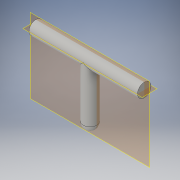
# Autodesk Inventor part: camPost
Saved by Autodesk Inventor 2016 (Build 200138000, 138)
## iProperties
Created: 2015-07-26
Part Number: camPost
Material: Generic
Document SubType Name: Modeling
Designer: steele
Density: 1 g/cm^3
Appearance: Default
Author: steele
Autodesk Inventor part; units mm, degrees
ref_plane "YZ Plane" through (0, 0, 0) normal (1, 0, 0) x (0, 1, 0)
sketch "Sketch1" plane through (0, 0, 0) normal (1, 0, 0) x (0, 1, 0)
  circle A0 centre (0, 0) radius 3.175
  dimension "postHoleDiam" = 6.35
  constraints: 1 centre point, 1 coincident
  measures "postHoleDiam" diameter of A0
extrude "Extrusion1" add sketch "Sketch1" along normal mid plane 50.8
sketch "Sketch3" plane through (0, 0, 0) normal (0, 1, 0) x (-1, 0, 0)
  circle A0 centre (0, 0) radius 3.175
  line L0 (25.4, 3.175) -> (-25.4, 3.175) projected
  constraints: 1 centre point, 1 coincident, 1 tangent
extrude "Extrusion2" add sketch "Sketch3" against normal blind 25.4
ref_plane "Work Plane1" through (0, -31.75, 0) normal (0, -1, 0) x (1, 0, 0)
sketch "Sketch5" plane through (0, 0, 0) normal (0, 0, 1) x (1, 0, 0)
  line L0 (-3.175, -25.4) -> (3.175, -25.4) projected
  arc A0 (-3.175, -25.4) -> (0, -28.575) centre (0, -25.4) ccw
  line L1 (0, -25.4) -> (0, -28.575)
  line L2 (-3.175, -25.4) -> (0, -25.4)
  point P0 (0, 0)
  constraints: 6 end point, 2 point on circle, 1 centre point, 1 horizontal, 1 midpoint
revolve "Revolution1" add sketch "Sketch5" angle 360 about axis through (0, -25.4, 0) along (0, -1, 0)
equation "\"postHoleDiam\" = hopperHoleDiam"
equation "\"camDiam\" = 6.35"
equation "\"hopperHoleDiam\" = 6.35"
body "Solid1"
